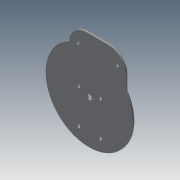
# Autodesk Inventor part: otocny_kruh1
Saved by Autodesk Inventor 2013 (Build 170138000, 138)
## iProperties
Created: 2013-01-26
Part Number: otocny_kruh1
Material: Generic
Document SubType Name: Modeling
Designer: idle-rug
Density: 1 g/cm^3
Author: idle-rug
Autodesk Inventor part; units mm, degrees
ref_plane "YZ Plane" through (0, 0, 0) normal (1, 0, 0) x (0, 1, 0)
ref_plane "XZ Plane" through (0, 0, 0) normal (0, 1, 0) x (-1, 0, 0)
ref_plane "XY Plane" through (0, 0, 0) normal (0, 0, 1) x (1, 0, 0)
sketch "Sketch1" plane through (0, 0, 0) normal (0, 1, 0) x (-1, 0, 0)
  circle A0 centre (0, 0) radius 50
  constraints: 1 centre point, 1 coincident
extrude "Extrusion1" add sketch "Sketch1" along normal blind 2
sketch "Sketch2" plane through (0, 0, 0) normal (0, -1, 0) x (1, 0, 0)
  circle A0 centre (0, 0) radius 50 projected
  circle A1 centre (0, 0) radius 3
  dimension "d3" = 6
  constraints: 1 centre point, 1 coincident
  measures "d3" diameter of A1
extrude "Extrusion2" cut sketch "Sketch2" against normal blind 2 contours A1
sketch "Sketch3" plane through (0, 0, 0) normal (0, -1, 0) x (1, 0, 0)
  circle A0 centre (0, 0) radius 50 projected
  circle A1 centre (0, 0) radius 11.5
  circle A2 centre (0, 0) radius 20
  circle A3 centre (0, 11.5) radius 2
  circle A4 centre (11.5, 0) radius 2
  circle A5 centre (-11.5, 0) radius 2
  circle A6 centre (0, -11.5) radius 2
  dimension "d15" = 23
  dimension "d16" = 40
  dimension "d17" = 4
  dimension "d18" = 4
  dimension "d19" = 4
  dimension "d20" = 4
  constraints: 6 centre point, 4 point on circle, 2 coincident
  measures "d15" diameter of A1
  measures "d16" diameter of A2
  measures "d17" diameter of A3
  measures "d18" diameter of A4
  measures "d19" diameter of A5
  measures "d20" diameter of A6
extrude "Extrusion3" cut sketch "Sketch3" against normal blind 2 contours A1 A4 | A1 A4 | A3 A1 | A1 A3 | A6 A1 | A1 A6 | A5 A1 | A1 A5
sketch "Sketch4" plane through (0, 0, 0) normal (0, -1, 0) x (1, 0, 0)
  circle A0 centre (0, -11.5) radius 2 projected
  circle A1 centre (11.5, 0) radius 2 projected
  circle A2 centre (0, 11.5) radius 2 projected
  circle A3 centre (-11.5, 0) radius 2 projected
extrude "Extrusion4" add sketch "Sketch4" against normal blind 2
sketch "Sketch5" plane through (0, 2, 0) normal (0, 1, 0) x (1, 0, 0)
  circle A0 centre (0, 0) radius 50 projected
  circle A1 centre (0, 0) radius 13.75
  circle A2 centre (0, 13.75) radius 2
  circle A3 centre (13.75, 0) radius 2
  circle A4 centre (0, -13.75) radius 2
  circle A5 centre (-13.75, 0) radius 2
  dimension "d25" = 27.5
  dimension "d26" = 4
  dimension "d27" = 4
  dimension "d28" = 4
  dimension "d29" = 4
  constraints: 5 centre point, 4 point on circle, 1 coincident
  measures "d25" diameter of A1
  measures "d26" diameter of A2
  measures "d27" diameter of A3
  measures "d28" diameter of A4
  measures "d29" diameter of A5
extrude "Extrusion5" cut sketch "Sketch5" against normal blind 2 contours A1 A3 | A1 A3 | A2 A1 | A1 A2 | A4 A1 | A1 A4 | A5 A1 | A1 A5
sketch "Sketch6" plane through (0, 0, 0) normal (0, -1, 0) x (1, 0, 0)
  line L0 (0, 0) -> (0, 63.2)
  line L1 (0, 63.2) -> (41.9, 63.2)
  line L2 (41.9, 63.2) -> (41.9, 27.2835)
  line L3 (0, 63.2) -> (-23.1, 63.2)
  line L4 (-23.1, 63.2) -> (-23.1, 44.344)
  arc A0 (41.9, 27.2835) -> (-23.1, 44.344) centre (0, 0) ccw
  arc A1 (41.9, 27.2835) -> (-23.1, 44.344) centre (0, 0) ccw
  line L5 (41.9, 27.2835) -> (41.9, 63.2)
  line L6 (41.9, 63.2) -> (-23.1, 63.2)
  line L7 (-23.1, 44.344) -> (-23.1, 63.2)
  dimension "d32" = 63.2
  dimension "d33" = 41.9
  dimension "d34" = 23.1
  constraints: 16 end point, 5 perpendicular, 4 point on circle, 2 centre point, 2 collinear, 1 vertical
  measures "d32" distance of L0.start L0.end
  measures "d33" distance of L0.end L1.end
  measures "d34" distance of L0.end L3.end
extrude "Extrusion6" add sketch "Sketch6" against normal blind 2
sketch "Sketch7" plane through (0, 0, 0) normal (0, -1, 0) x (1, 0, 0)
  line L0 (41.9, 27.2835) -> (41.9, 63.2) projected
  line L1 (-23.1, 63.2) -> (41.9, 63.2)
  line L2 (41.9, 63.2) -> (41.9, 32.6)
  line L3 (41.9, 32.6) -> (-23.1, 32.6)
  line L4 (-23.1, 32.6) -> (-23.1, 63.2)
  line L5 (41.9, 32.6) -> (31.9, 32.6)
  line L6 (31.9, 32.6) -> (31.9, 47.9)
  line L7 (31.9, 47.9) -> (41.9, 47.9)
  line L8 (41.9, 47.9) -> (41.9, 32.6)
  line L9 (-23.1, 32.6) -> (-13.1, 32.6)
  line L10 (-13.1, 32.6) -> (-13.1, 47.9)
  line L11 (-13.1, 47.9) -> (-23.1, 47.9)
  line L12 (-23.1, 47.9) -> (-23.1, 32.6)
  circle A0 centre (31.9, 47.9) radius 2
  circle A1 centre (-13.1, 47.9) radius 2
  dimension "d37" = 30.6
  dimension "d38" = 10
  dimension "d39" = 15.3
  dimension "d40" = 10
  dimension "d41" = 15.3
  dimension "d42" = 4
  dimension "d43" = 4
  constraints: 24 end point, 6 parallel, 3 horizontal, 3 perpendicular, 2 centre point, 2 coincident, 1 point on line
  measures "d37" distance of L1.end L2.end
  measures "d38" distance of L6.end L7.end
  measures "d39" distance of L5.end L6.end
  measures "d40" distance of L11.end L10.end
  measures "d41" distance of L10.end L9.end
  measures "d42" diameter of A0
  measures "d43" diameter of A1
extrude "Extrusion7" cut sketch "Sketch7" against normal blind 2 contours A0 L6 L7 | L7 L6 A0 | A1 L11 L10 | L10 L11 A1
fillet "Fillet1" radius 20 2 edges at (41.9, 1, 63.2) (-23.1, 1, 63.2)
sketch "Sketch9" plane through (0, 0, 0) normal (0, -1, 0) x (1, 0, 0)
  circle A0 centre (-13.75, 0) radius 2 projected
  circle A1 centre (13.75, 0) radius 2 projected
  circle A2 centre (0, -13.75) radius 2 projected
  circle A3 centre (0, 13.75) radius 2 projected
  circle A4 centre (0, 0) radius 3 projected
extrude "Extrusion8" add sketch "Sketch9" against normal blind 2
sketch "Sketch10" plane through (0, 2, 0) normal (0, 1, 0) x (1, 0, 0)
  circle A0 centre (12.5, 35) radius 2
  circle A1 centre (-12.5, 35) radius 2
  circle A2 centre (12.5, -5) radius 2
  circle A3 centre (-12.5, -5) radius 2
  dimension "d55" = 4
  dimension "d56" = 4
  dimension "d59" = 4
  dimension "d60" = 4
  constraints: 4 centre point
  measures "d55" diameter of A0
  measures "d56" diameter of A1
  measures "d59" diameter of A2
  measures "d60" diameter of A3
extrude "Extrusion9" cut sketch "Sketch10" against normal blind 2
sketch "Sketch11" plane through (0, 2, 0) normal (0, 1, 0) x (1, 0, 0)
  arc A0 (41.9, -27.2835) -> (-23.1, -44.344) centre (0, 0) ccw projected
  circle A1 centre (0, 0) radius 3
  dimension "d63" = 6
  constraints: 1 centre point, 1 coincident
  measures "d63" diameter of A1
extrude "Extrusion10" cut sketch "Sketch11" against normal blind 2
body "Solid1"
